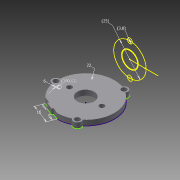
# Autodesk Inventor part: ReduktorLemez
Saved by Autodesk Inventor 2015 (Build 190159000, 159)
## iProperties
Created: 2014-09-27
Part Number: ReduktorLemez
Material: Generic
Document SubType Name: Modeling
Designer: laca
Density: 1 g/cm^3
Appearance: Default
Mass: 5.44083 g
Surface Area: 37.3446 cm^2
Volume: 5.44083 cm^3
Author: laca
Autodesk Inventor part; units mm, degrees
ref_plane "YZ Plane" through (0, 0, 0) normal (1, 0, 0) x (0, 1, 0)
ref_plane "XZ Plane" through (0, 0, 0) normal (0, 1, 0) x (-1, 0, 0)
ref_plane "XY Plane" through (0, 0, 0) normal (0, 0, 1) x (1, 0, 0)
sketch "Sketch1" plane through (0, 0, 0) normal (0, 1, 0) x (-1, 0, 0)
  arc A0 (21.9195, -1.8799) -> (21.6133, 4.1068) centre (21.8945, 1.12) ccw
  arc A1 (-9.3318, 19.9228) -> (-14.3633, 16.6642) centre (-11.9173, 18.4012) ccw
  arc A2 (-12.5878, -18.043) -> (-7.25, -20.7711) centre (-9.9773, -19.5212) ccw
  line L0 (4.6577, 20.1818) -> (5.0644, 21.2236)
  line L1 (10.6536, 19.0418) -> (10.247, 18)
  line L2 (5.0644, 21.2236) -> (10.6536, 19.0418)
  line L3 (14.9047, 16.1818) -> (10.247, 18)
  line L4 (4.6577, 20.1818) -> (0, 22)
  line L5 (21.8945, 1.12) -> (19.0999, 2.211)
  arc A3 (-14.3633, 16.6642) -> (-12.5878, -18.043) centre (0, 0) ccw
  arc A4 (-7.25, -20.7711) -> (21.9195, -1.8799) centre (0, 0) ccw
  arc A5 (21.6133, 4.1068) -> (14.9047, 16.1818) centre (0, 0) ccw
  arc A6 (0, 22) -> (-9.3318, 19.9228) centre (0, 0) ccw
  dimension "d1" = 6
  dimension "d4" = 360
  dimension "d7" = 16
  dimension "d8" = 5
  dimension "d9" = 5
  dimension "d18" = 22
  constraints: 15 point on circle, 12 end point, 7 centre point, 4 perpendicular, 3 parallel, 1 coincident, 1 collinear, 13 other
  measures "d1" diameter of A0
  measures "d7" distance of L3.start L4.end
  measures "d8" distance from line of L0 L4.end
  measures "d9" distance from line of L3.start L1
  measures "d18" radius of A4
extrude "Extrusion1" add sketch "Sketch1" along normal blind 4
sketch "Sketch2" plane through (0, 4, 0) normal (0, 1, 0) x (1, 0, 0)
  arc A0 (-21.9195, 1.8799) -> (-21.6133, -4.1068) centre (-21.8945, -1.12) ccw projected
  circle A1 centre (-21.8945, -1.12) radius 2
  arc A2 (12.5878, 18.043) -> (7.25, 20.7711) centre (9.9773, 19.5212) ccw projected
  circle A3 centre (9.9773, 19.5212) radius 2
  arc A4 (9.3318, -19.9228) -> (14.3633, -16.6642) centre (11.9173, -18.4012) ccw projected
  circle A5 centre (11.9173, -18.4012) radius 2
  circle A6 centre (0, 0) radius 6.5
  dimension "d12" = 4
  dimension "d13" = 4
  dimension "d14" = 4
  dimension "d15" = 13
  constraints: 4 centre point, 4 coincident
  measures "d12" diameter of A1
  measures "d13" diameter of A3
  measures "d14" diameter of A5
  measures "d15" diameter of A6
extrude "Extrusion2" cut sketch "Sketch2" against normal through all
derived "Haz.ipt"
sketch "Sketch3" plane through (-11.8815, 0, -45.8133) normal (0, 0, -1) x (-1, 0, 0)
  circle A0 centre (0, 0) radius 6.5
  circle A1 centre (0, 0) radius 6
  circle A2 centre (0, 0) radius 12.5
  circle A3 centre (0, 12.5) radius 1.9
  circle A4 centre (0, -12.5) radius 1.9
  line L0 (0, 0) -> (-21.7112, 0)
  point P0 (-11.8815, 0)
  dimension "d20" = 25
  dimension "d21" = 3.8
  measures "d21" diameter of A3
sketch "Sketch4" plane through (0, 4, 0) normal (0, 1, 0) x (1, 0, 0)
  circle A0 centre (0, 0) radius 12.5
  circle A1 centre (-12.5, 0) radius 1.9
  circle A2 centre (12.5, 0) radius 1.9
  dimension "d22" = 25
  dimension "d23" = 3.8
  dimension "d24" = 3.8
  constraints: 3 centre point, 2 point on circle, 1 coincident
  measures "d22" diameter of A0
  measures "d23" diameter of A1
  measures "d24" diameter of A2
extrude "Extrusion3" cut sketch "Sketch4" against normal through all contours A0 A2 | A0 A2 | A1 A0 | A0 A1
equation "\"d22\" = d20"
equation "\"d23\" = d21"
equation "\"d24\" = d21"
body "Solid1"
